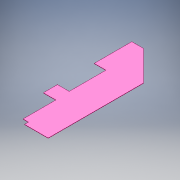
# Autodesk Inventor part: Gearbox-Side Cover Part 2
Saved by Autodesk Inventor 2018 (Build 220112000, 112)
## iProperties
Created: 2018-08-07
Part Number: Gearbox-Side Cover Part 2
Material: Steel
Document SubType Name: Modeling
Designer: P301319
Density: 7.85 g/cm^3
Appearance: Pink
Author: P301319
Autodesk Inventor part; units mm, degrees
ref_plane "YZ Plane" through (0, 0, 0) normal (1, 0, 0) x (0, 1, 0)
ref_plane "XZ Plane" through (0, 0, 0) normal (0, 1, 0) x (-1, 0, 0)
ref_plane "XY Plane" through (0, 0, 0) normal (0, 0, 1) x (1, 0, 0)
sketch "Sketch1" plane through (0, 0, 0) normal (0, 0, 1) x (1, 0, 0)
  line L0 (0, 0) -> (0, 240)
  line L1 (0, 0) -> (75, 0)
  line L2 (0, 240) -> (75, 240)
  line L3 (75, 240) -> (338.7516, 240) construction
  line L4 (75, 0) -> (75, -235)
  line L5 (75, -235) -> (0, -235)
  line L6 (0, -235) -> (0, -325)
  line L7 (0, -325) -> (80, -325)
  line L8 (80, -325) -> (80, -535)
  line L9 (80, -535) -> (115, -535)
  line L10 (115, -535) -> (115, -560)
  line L11 (115, -560) -> (265.9188, -560)
  line L12 (75, 240) -> (265.9188, 49.0812)
  line L13 (75, 240) -> (345, 240) construction
  line L14 (265.9188, 49.0812) -> (265.9188, -560)
  dimension "d0" = 240
  dimension "d1" = 75
  dimension "d4" = 235
  dimension "d5" = 75
  dimension "d6" = 90
  dimension "d7" = 80
  dimension "d8" = 210
  dimension "d9" = 35
  dimension "d10" = 25
  dimension "d16" = 75
  dimension "d17" = 270
  dimension "d18" = 45
  constraints: 30 end point, 7 horizontal, 5 vertical, 2 perpendicular, 1 equal length
  measures "d0" distance of L0.start L0.end
  measures "d1" distance of L0.start L1.end
  measures "d4" distance of L1.end L4.end
  measures "d5" distance of L4.end L5.end
  measures "d6" distance of L5.end L6.end
  measures "d7" distance of L6.end L7.end
  measures "d8" distance of L7.end L8.end
  measures "d9" distance of L8.end L9.end
  measures "d10" distance of L9.end L10.end
  measures "d16" distance of L0.end L2.end
  measures "d17" distance of L2.end L12.end
  measures "d18" angle of L12 L13
extrude "Extrusion1" add sketch "Sketch1" along normal blind 1.6
equation "\"d5\" = d1"
body "Solid1"
